brazo armado (Autodesk Fusion 360 archive; units mm, degrees)
design "brazos"
Autodesk Fusion 360 part; units mm, degrees
sketch "Sketch1" plane through (0, 0, 0) normal (1, 0, 0) x (0, 1, 0)
  circle A0 centre (0, 0) radius 5
  line L0 (0, 5) -> (80, 5)
  line L1 (0, -5) -> (80, -5)
  circle A1 centre (80, 0) radius 5
  dimension "d1" = 10
  dimension "d2" = 80
  constraint coincident A0.centre origin
  constraint coincident A0 L0.start
  constraint horizontal L0
  constraint coincident A0 L1.start
  constraint tangent A0 L1
  constraint parallel L0 L1
  constraint coincident L0.end A1
  constraint tangent L0 A1
  measures "d1" diameter of A0
  measures "d2" distance of L0.start L0.end
extrude "Extrude1" add sketch "Sketch1" along normal blind 4
sketch "Sketch2" plane through (4, 0, 0) normal (1, 0, 0) x (0, 1, 0)
  arc A0 (0, 5) -> (0, -5) centre (0, 0) ccw
  line L0 (0, -5) -> (80, -5)
  arc A1 (80, -5) -> (80, 5) centre (80, 0) ccw
  line L1 (80, 5) -> (0, 5)
  circle A2 centre (0, 0) radius 2
  circle A3 centre (80, 0) radius 2
  dimension "d5" = 4
  dimension "d6" = 4
  constraint coincident A0.centre A2.centre
  constraint concentric A1 A3
  measures "d5" diameter of A2
  measures "d6" diameter of A3
extrude "Extrude2" cut sketch "Sketch2" against normal blind 20 contours A2 | A3
sketch "Sketch3" plane through (4, 0, 0) normal (1, 0, 0) x (0, 1, 0)
  circle A0 centre (0, 0) radius 2
  circle A1 centre (80, 0) radius 2
  arc A2 (0, 5) -> (0, -5) centre (0, 0) ccw
  line L0 (0, -5) -> (80, -5)
  arc A3 (80, -5) -> (80, 5) centre (80, 0) ccw
  line L1 (80, 5) -> (0, 5)
  circle A4 centre (40, 0) radius 2
  dimension "d9" = 4
  measures "d9" diameter of A4
extrude "Extrude3" cut sketch "Sketch3" against normal blind 20 contours A4
sketch "Sketch4" plane through (0, 0, 0) normal (0, 0, 1) x (1, 0, 0)
sketch "Sketch5" plane through (4, 0, 0) normal (1, 0, 0) x (0, 1, 0)
  circle A0 centre (40, 0) radius 2
  circle A1 centre (0, 0) radius 2
  circle A2 centre (80, 0) radius 2
  arc A3 (0, 5) -> (0, -5) centre (0, 0) ccw
  line L0 (0, -5) -> (80, -5)
  arc A4 (80, -5) -> (80, 5) centre (80, 0) ccw
  line L1 (80, 5) -> (0, 5)

design "Untitled" references "eje", "brazos", "agarre de tuerca", "Untitled", "guia", "varilla roscada", "soporte motores v1 horus"
Autodesk Fusion 360 part; units mm, degrees
sketch "Sketch1" plane through (0, 0, 0) normal (1, 0, 0) x (0, 1, 0)
  line L0 (0, 0) -> (42, 0)
  line L1 (42, 0) -> (42, 42)
  line L2 (42, 42) -> (0, 42)
  line L3 (0, 42) -> (0, 0)
  dimension "d1" = 42
  dimension "d2" = 42
  constraint horizontal L0
  constraint vertical L1
  constraint horizontal L2
  constraint vertical L3
  constraint coincident L0.start L3.end
  measures "d1" distance of L0.start L0.end
  measures "d2" distance of L0.start L2.end
extrude "Extrude1" add sketch "Sketch1" along normal blind 30
sketch "Sketch2" plane through (30, 0, 0) normal (1, 0, 0) x (0, 1, 0)
  line L0 (0, 42) -> (0, 0)
  line L1 (0, 0) -> (42, 0)
  line L2 (42, 0) -> (42, 42)
  line L3 (42, 42) -> (0, 42)
  line L4 (42, 0) -> (0, 0)
  line L5 (0, 0) -> (0, 42)
  line L6 (0, 42) -> (42, 42)
  line L7 (42, 42) -> (42, 0)
  line L8 (42, 0) -> (0, 42) construction
  line L9 (0, 0) -> (42, 42) construction
  point P0 (21, 21)
  constraint horizontal L4
  constraint perpendicular L4 L5
  constraint parallel L4 L6
  constraint parallel L5 L7
  constraint coincident L8 P0
  constraint coincident L9 P0
  constraint coincident L1.end L2.start
  constraint coincident L0.start L3.end
extrude "Extrude2" add 1 faces at (30, 28, 28) along direction (1, 0, 0) blind 1
sketch "Sketch3" plane through (31, 0, 0) normal (1, 0, 0) x (0, 1, 0)
  line L0 (0, 42) -> (0, 0)
  line L1 (0, 0) -> (42, 0)
  line L2 (42, 0) -> (42, 42)
  line L3 (42, 42) -> (0, 42)
  circle A0 centre (21, 21) radius 5
  dimension "d7" = 10
  measures "d7" diameter of A0
extrude "Extrude3" cut sketch "Sketch3" against normal blind 2 contours A0
sketch "Sketch5" plane through (29, 0, 0) normal (1, 0, 0) x (0, 1, 0)
  circle A0 centre (21, 21) radius 5
  circle A1 centre (21, 21) radius 2.5
  dimension "d11" = 5
  constraint concentric A0 A1
  measures "d11" diameter of A1
extrude "Extrude4" add sketch "Sketch5" along normal blind 13 contours A1
sketch "Sketch6" plane through (42, 0, 0) normal (1, 0, 0) x (0, 1, 0)
  circle A0 centre (21, 21) radius 2.5
  circle A1 centre (21, 21) radius 5
  dimension "d14" = 10
  constraint concentric A0 A1
  measures "d14" diameter of A1
extrude "Extrude5" add sketch "Sketch6" along normal blind 13 contours A0 | A1
sketch "Sketch7" plane through (31, 0, 0) normal (1, 0, 0) x (0, 1, 0)
  circle A0 centre (21, 21) radius 5
  line L0 (0, 42) -> (0, 0)
  line L1 (0, 0) -> (42, 0)
  line L2 (42, 0) -> (42, 42)
  line L3 (42, 42) -> (0, 42)
  line L4 (42, 21) -> (42, 28.5)
  line L5 (42, 21) -> (42, 13.5)
  line L6 (42, 21) -> (50, 21)
  line L7 (0, 28.4982) -> (0, 21)
  line L8 (0, 13.5018) -> (0, 21)
  line L9 (0, 21) -> (-8, 21)
  circle A1 centre (-8, 21) radius 2.5
  circle A2 centre (50, 21) radius 2.5
  line L10 (-9.3249, 23.12) -> (0, 28.4982)
  line L11 (-9.3248, 18.8799) -> (0, 13.5018)
  line L12 (42, 13.5) -> (51.249, 18.8344)
  line L13 (51.249, 23.1656) -> (42, 28.5)
  dimension "d17" = 7.5
  dimension "d18" = 7.5
  dimension "d19" = 8
  dimension "d20" = 8
  dimension "d21" = 5
  dimension "d22" = 5
  constraint midpoint L2 L4.start
  constraint perpendicular L3 L4
  constraint parallel L2 L5
  constraint perpendicular L4 L6
  constraint coincident L0 L7.start
  constraint midpoint L0 L7.end
  constraint parallel L0 L7
  constraint coincident L0 L8.start
  constraint parallel L0 L8
  constraint perpendicular L7 L9
  constraint coincident L9.end A1.centre
  constraint coincident L6.end A2.centre
  constraint coincident A1 L10.start
  constraint coincident A1 L11.start
  constraint coincident A2 L12.end
  constraint parallel L10 L12
  constraint coincident A2 L13.start
  constraint parallel L11 L13
  measures "d17" distance of L4.start L4.end
  measures "d18" distance of L4.start L5.end
  measures "d19" distance of L4.start L6.end
  measures "d20" distance of L7.end L9.end
  measures "d21" diameter of A1
  measures "d22" diameter of A2
extrude "Extrude6" add sketch "Sketch7" against normal blind 1 contours L0 L7 L9 A1 L10 | L0 L8 L9 A1 L11 | A1 L10 L11 | L2 L4 L6 A2 L13 | L2 L5 L6 A2 L12 | A2
sketch "Sketch8" plane through (31, 0, 0) normal (1, 0, 0) x (0, 1, 0)
  circle A0 centre (21, 21) radius 5
  line L0 (0, 42) -> (0, 28.4982)
  line L1 (0, 28.4982) -> (-9.3249, 23.12)
  arc A1 (-9.3249, 23.12) -> (-9.3248, 18.8799) centre (-8, 21) ccw
  line L2 (-9.3248, 18.8799) -> (0, 13.5018)
  line L3 (0, 13.5018) -> (0, 0)
  line L4 (0, 0) -> (42, 0)
  line L5 (42, 0) -> (42, 13.5)
  line L6 (42, 13.5) -> (51.249, 18.8344)
  arc A2 (51.249, 18.8344) -> (51.249, 23.1656) centre (50, 21) ccw
  line L7 (51.249, 23.1656) -> (42, 28.5)
  line L8 (42, 28.5) -> (42, 42)
  line L9 (42, 42) -> (0, 42)
  circle A3 centre (-8, 21) radius 1.5
  circle A4 centre (50, 21) radius 1.5
  dimension "d25" = 3
  dimension "d26" = 3
  constraint concentric A1 A3
  constraint concentric A2 A4
  measures "d25" diameter of A3
  measures "d26" diameter of A4
extrude "Extrude7" cut sketch "Sketch8" against normal blind 5 contours A3 | A4
fillet "Fillet1" radius 7.5 4 edges at (15.5, 42, 42) (15.5, 0, 42) (15.5, 0, 0) (15.5, 42, 0)

design "guia"
Autodesk Fusion 360 part; units mm, degrees
sketch "Sketch1" plane through (0, 0, 0) normal (1, 0, 0) x (0, 1, 0)
  line L0 (0, 0) -> (100, 0)
  line L1 (100, 0) -> (100, 15)
  line L2 (100, 15) -> (0, 15)
  line L3 (0, 15) -> (0, 0)
  dimension "d1" = 100
  dimension "d2" = 15
  constraint horizontal L0
  constraint vertical L1
  constraint horizontal L2
  constraint vertical L3
  constraint coincident L0.start L3.end
  measures "d1" distance of L0.start L0.end
  measures "d2" distance of L0.start L2.end
extrude "Extrude1" add sketch "Sketch1" along normal blind 6
sketch "Sketch2" plane through (6, 0, 0) normal (1, 0, 0) x (0, 1, 0)
  line L0 (0, 15) -> (0, 0)
  line L1 (0, 0) -> (100, 0)
  line L2 (100, 0) -> (100, 15)
  line L3 (100, 15) -> (0, 15)
  circle A0 centre (6, 7.5) radius 4
  circle A1 centre (94, 7.5) radius 4
  line L4 (6, 11.5) -> (94, 11.5)
  line L5 (94, 3.5) -> (6, 3.5)
  dimension "d5" = 8
  dimension "d6" = 6
  dimension "d7" = 8
  dimension "d8" = 6
  constraint coincident A0 L4.start
  constraint coincident A1 L4.end
  constraint tangent A1 L4
  constraint perpendicular L2 L4
  constraint coincident A1 L5.start
  constraint coincident A0 L5.end
  constraint tangent A0 L5
  constraint parallel L1 L5
  measures "d5" diameter of A0
  measures "d6" distance of L0 A0.centre
  measures "d7" diameter of A1
  measures "d8" distance of L2 A1.centre
extrude "Extrude2" cut sketch "Sketch2" against normal blind 20 contours A0 | A0 A1 L4 L5 | A1
sketch "Sketch3" plane through (0, 0, 0) normal (-1, 0, 0) x (0, -1, 0)
  line L0 (-6, 3.5) -> (-94, 3.5)
  arc A0 (-94, 11.5) -> (-94, 3.5) centre (-94, 7.5) ccw
  line L1 (-94, 11.5) -> (-6, 11.5)
  arc A1 (-6, 3.5) -> (-6, 11.5) centre (-6, 7.5) ccw
  line L2 (0, 0) -> (0, 15)
  line L3 (0, 15) -> (-100, 15)
  line L4 (-100, 15) -> (-100, 0)
  line L5 (-100, 0) -> (0, 0)
sketch "Sketch4" plane through (0, 50, 7.5) normal (-1, 0, 0) x (0, -1, 0)
sketch "Sketch5" plane through (0, 0, 0) normal (0, 0, -1) x (1, 0, 0)
  line L0 (0, 0) -> (0, -100)
  line L1 (0, -100) -> (6, -100)
  line L2 (6, -100) -> (6, 0)
  line L3 (6, 0) -> (0, 0)
  line L4 (0, -100) -> (-5, -100)
  line L5 (-5, -100) -> (-5, -95)
  line L6 (-5, -95) -> (0, -95)
  line L7 (0, -95) -> (0, -100)
  line L8 (0, 0) -> (-5, 0)
  line L9 (-5, 0) -> (-5, -5)
  line L10 (-5, -5) -> (0, -5)
  line L11 (0, -5) -> (0, 0)
  dimension "d11" = 5
  dimension "d12" = 5
  dimension "d13" = 5
  dimension "d14" = 5
  constraint horizontal L4
  constraint vertical L5
  constraint horizontal L6
  constraint vertical L7
  constraint coincident L0.end L1.start
  constraint horizontal L8
  constraint vertical L9
  constraint horizontal L10
  constraint vertical L11
  constraint coincident L0.start L3.end
  measures "d11" distance of L0.end L4.end
  measures "d12" distance of L0.end L6.end
  measures "d13" distance of L0.start L8.end
  measures "d14" distance of L0.start L10.end
extrude "Extrude3" add sketch "Sketch5" against normal blind 3 contours L0 L8 L9 L10 L11 | L0 L4 L5 L6 L7
sketch "Sketch6" plane through (0, 0, 3) normal (0, 0, 1) x (-1, 0, 0)
  line L0 (5, -95) -> (0, -95)
  line L1 (0, -95) -> (0, -100)
  line L2 (0, -100) -> (5, -100)
  line L3 (5, -100) -> (5, -95)
  circle A0 centre (2.5, -97.5) radius 2
  dimension "d17" = 4
  measures "d17" diameter of A0
extrude "Extrude4" cut sketch "Sketch6" against normal blind 6 contours A0
sketch "Sketch7" plane through (0, 0, 0) normal (-1, 0, 0) x (0, -1, 0)
sketch "Sketch8" plane through (0, 0, 3) normal (0, 0, 1) x (-1, 0, 0)
  line L0 (0, 0) -> (0, -5)
  line L1 (0, -5) -> (5, -5)
  line L2 (5, -5) -> (5, 0)
  line L3 (5, 0) -> (0, 0)
  circle A0 centre (2.5, -2.5) radius 2
  dimension "d20" = 4
  measures "d20" diameter of A0
extrude "Extrude5" cut sketch "Sketch8" against normal blind 9 contours A0

design "eje"
Autodesk Fusion 360 part; units mm, degrees
sketch "Sketch1" plane through (0, 0, 0) normal (1, 0, 0) x (0, 1, 0)
  circle A0 centre (0, 0) radius 2
  dimension "d1" = 4
  constraint coincident A0.centre origin
  measures "d1" diameter of A0
extrude "Extrude1" add sketch "Sketch1" against normal blind 40

design "agarre de tuerca"
Autodesk Fusion 360 part; units mm, degrees
sketch "Sketch1" plane through (0, 0, 0) normal (1, 0, 0) x (0, 1, 0)
  line L0 (0, 0) -> (12, 0)
  line L1 (12, 0) -> (12, 10)
  line L2 (12, 10) -> (0, 10)
  line L3 (0, 10) -> (0, 0)
  circle A0 centre (8, 5) radius 2
  dimension "d3" = 12
  dimension "d4" = 4
  constraint horizontal L0
  constraint vertical L1
  constraint horizontal L2
  constraint vertical L3
  constraint coincident L0.start L3.end
  measures "d3" distance of L1 L3
  measures "d4" diameter of A0
extrude "Extrude1" add sketch "Sketch1" along normal blind 4 contours L0 L1 L2 L3 | A0 makes body 1
extrude "Extrude2" add sketch "Sketch1" along normal blind 4 separate body makes body 2
extrude "Extrude4" cut sketch "Sketch1" along normal blind 125 contours A0 bodies 1
sketch "Sketch3" plane through (0, 6, 5) normal (1, 0, 0) x (0, 1, 0)
  line L0 (-6, 5) -> (-2, 5)
  line L1 (-2, 5) -> (-2, -5)
  line L2 (-6, -5) -> (-6, 5)
  line L3 (-2, -5) -> (-6, -5)
  constraint horizontal L0
  constraint perpendicular L0 L1
  constraint perpendicular L0 L2
  constraint perpendicular L2 L3
extrude "Extrude5" add sketch "Sketch3" along normal blind 80 bodies 1 2
sketch "Sketch4" plane through (0, 4, 0) normal (0, 1, 0) x (-1, 0, 0)
  line L0 (-4, 0) -> (-4, 10)
  line L1 (-4, 10) -> (-80, 10)
  line L2 (-80, 10) -> (-80, 0)
  line L3 (-80, 0) -> (-4, 0)
  circle A0 centre (-42, 5) radius 2
extrude "Extrude6" cut sketch "Sketch4" against normal blind 14 contours A0 bodies 1
sketch "Sketch5" plane through (0, 0, 10) normal (0, 0, 1) x (-1, 0, 0)
  line L0 (-4, -4) -> (-4, -12)
  line L1 (-4, -12) -> (0, -12)
  line L2 (0, -12) -> (0, 0)
  line L3 (0, 0) -> (-80, 0)
  line L4 (-80, 0) -> (-80, -4)
  line L5 (-80, -4) -> (-4, -4)
  line L6 (-80, 0) -> (-84, 0)
  line L7 (-84, 0) -> (-84, -12)
  line L8 (-84, -12) -> (-80, -12)
  line L9 (-80, -12) -> (-80, 0)
  dimension "d15" = 4
  constraint coincident L3.end L4.start
  constraint perpendicular L4 L6
  constraint perpendicular L1 L7
  constraint perpendicular L7 L8
  constraint parallel L4 L9
  measures "d15" distance of L3.end L6.end
extrude "Extrude7" add sketch "Sketch5" against normal blind 10 contours L4 L6 L7 L8 L9 bodies 1
extrude "Extrude8" cut sketch "Sketch1" along normal blind 360 contours A0 bodies 1
sketch "Sketch6" plane through (0, 4, 0) normal (0, 1, 0) x (-1, 0, 0)
  circle A0 centre (-42, 5) radius 2
  line L0 (-4, 0) -> (-4, 10)
  line L1 (-4, 10) -> (-80, 10)
  line L2 (-80, 10) -> (-80, 0)
  line L3 (-80, 0) -> (-4, 0)
  circle A1 centre (-42, 5) radius 5
  line L4 (-42, 5) -> (-40, 5)
  line L5 (-37, 5) -> (-47, 5)
  line L6 (-37, 5) -> (-37.5116, 6.9335)
  line L7 (-47, 5) -> (-46.4882, 6.9334)
  line L8 (-47, 5) -> (-46.6078, 3.0388)
  line L9 (-37, 5) -> (-37.5177, 3.0682)
  line L10 (-46.4882, 6.9334) -> (-80, 10)
  line L11 (-46.6078, 3.0388) -> (-80, 0)
  line L12 (-37.5116, 6.9335) -> (-4, 10)
  line L13 (-37.5177, 3.0682) -> (-4, 0)
  dimension "d20" = 2
  dimension "d21" = 2
  dimension "d22" = 2
  dimension "d23" = 2
  constraint concentric A0 A1
  constraint tangent L1 A1
  constraint coincident A0.centre A1.centre
  constraint coincident A0 L4.end
  constraint horizontal L4
  constraint coincident A1 L5.start
  constraint coincident A1 L5.end
  constraint parallel L4 L5
  constraint coincident L1.end L2.start
  constraint coincident L2.end L3.start
  constraint coincident L0.end L1.start
  constraint coincident L0.start L3.end
  measures "d20" distance of L5.start L6.end
  measures "d21" distance of L5.end L7.end
  measures "d22" distance of L5.end L8.end
  measures "d23" distance of L5.start L9.end
extrude "Extrude9" cut sketch "Sketch6" against normal blind 20 contours L1 A1 L12 | L3 A1 L13 | L1 A1 L10 | L3 A1 L8 L11 bodies 1
fillet "Fillet1" radius 2.5 4 edges at (0, 0, 5) (84, 0, 5) (80, 4, 5) (4, 4, 5) on bodies 1
